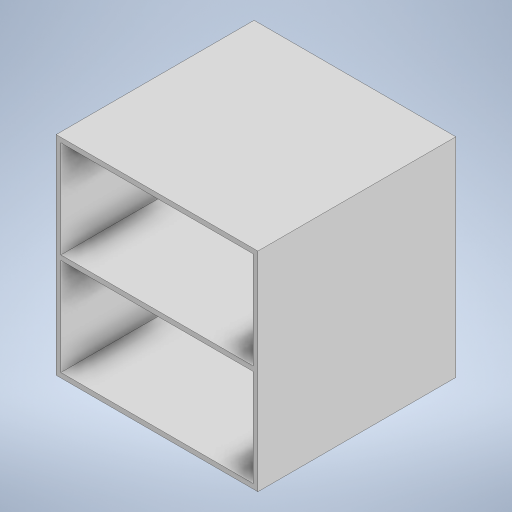
# Autodesk Inventor part: 10cmX10cmDrawerHolder
Saved by Autodesk Inventor 2024 (Build 280153000, 153)
## iProperties
Created: 2023-09-24
Part Number: 10cmX10cmDrawerHolder
Material: Generic
Document SubType Name: Modeling
Designer: Family2
Density: 1 g/cm^3
Appearance: Default
Mass: 166.626 g
Surface Area: 1294.46 cm^2
Volume: 166.626 cm^3
Author: Family2
Autodesk Inventor part; units mm, degrees
ref_plane "YZ Plane" through (0, 0, 0) normal (1, 0, 0) x (0, 1, 0)
ref_plane "XZ Plane" through (0, 0, 0) normal (0, 1, 0) x (-1, 0, 0)
ref_plane "XY Plane" through (0, 0, 0) normal (0, 0, 1) x (1, 0, 0)
sketch "Sketch1" plane through (0, 0, 0) normal (0, 0, 1) x (1, 0, 0)
  line L0 (0, 0) -> (106, 0)
  line L1 (0, 0) -> (0, -54.75)
  line L2 (106, 0) -> (106, -54.75)
  line L3 (0, -54.75) -> (106, -54.75) construction
  line L4 (0, -109.5) -> (106, -109.5)
  line L5 (0, -109.5) -> (0, -54.75)
  line L6 (106, -109.5) -> (106, -54.75)
  dimension "d0" = 106
  dimension "d1" = 54.75
  dimension "d6" = 54.75
  constraints: 14 end point, 2 symmetric about line, 2 vertical, 1 horizontal
  measures "d0" distance of L0.start L0.end
  measures "d1" distance of L0.start L1.end
  measures "d6" distance of L0.end L2.end
extrude "Extrusion3" add sketch "Sketch1" along normal blind 104
sketch "Sketch4" plane through (0, 0, 104) normal (0, 0, 1) x (1, 0, 0)
  line L0 (106, -109.5) -> (106, 0) construction
  line L1 (0, 0) -> (106, 0) construction
  line L2 (106, 0) -> (106, -54.75) construction
  line L3 (106, -54.75) -> (0, -54.75) construction
  line L4 (0, -54.75) -> (0, 0) construction
  line L5 (0, 0) -> (0, -109.5) construction
  line L6 (0, -109.5) -> (106, -109.5) construction
  line L7 (106, -109.5) -> (106, -54.75) construction
  line L8 (106, -54.75) -> (0, -54.75) construction
  line L9 (0, -54.75) -> (0, -109.5) construction
  line L10 (2.5, -53.5) -> (103.5, -53.5)
  line L11 (103.5, -53.5) -> (103.5, -2.5)
  line L12 (103.5, -2.5) -> (2.5, -2.5)
  line L13 (2.5, -2.5) -> (2.5, -53.5)
  line L14 (2.5, -56) -> (103.5, -56)
  line L15 (103.5, -56) -> (103.5, -107)
  line L16 (103.5, -107) -> (2.5, -107)
  line L17 (2.5, -107) -> (2.5, -56)
  line L18 (106, 0) -> (0, 0) projected
  line L19 (53, 0) -> (53, -109.5) construction
  dimension "d61" = 2.5
  dimension "d62" = 2.5
  dimension "d63" = 2.5
  dimension "d64" = 1.25
  dimension "d65" = 1.25
  dimension "d66" = 2.5
  dimension "d67" = 2.5
  dimension "d68" = 2.5
  constraints: 34 end point, 8 parallel, 4 horizontal, 4 perpendicular, 3 midpoint
  measures "d61" distance between parallel lines of L12 L1
  measures "d62" distance between parallel lines of L0 L11
  measures "d63" distance between parallel lines of L4 L13
  measures "d64" distance between parallel lines of L3 L10
  measures "d65" distance between parallel lines of L8 L14
  measures "d66" distance between parallel lines of L0 L15
  measures "d67" distance between parallel lines of L9 L17
  measures "d68" distance between parallel lines of L6 L16
extrude "Extrusion4" cut sketch "Sketch4" against normal blind 101
body "Solid3"
